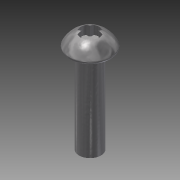
# Autodesk Inventor part: Screw
Saved by Autodesk Inventor 2015 (Build 190159000, 159)
## iProperties
Created: 2016-01-20
Part Number: Screw
Material: Generic
Document SubType Name: Modeling
Designer: Kyle
Density: 1 g/cm^3
Appearance: Galvanized
Author: Kyle
Autodesk Inventor part; units mm, degrees
ref_plane "YZ Plane" through (0, 0, 0) normal (1, 0, 0) x (0, 1, 0)
ref_plane "XZ Plane" through (0, 0, 0) normal (0, 1, 0) x (-1, 0, 0)
ref_plane "XY Plane" through (0, 0, 0) normal (0, 0, 1) x (1, 0, 0)
sketch "Sketch1" plane through (0, 0, 0) normal (0, 0, 1) x (1, 0, 0)
  line L0 (2.1581, 5.715) -> (1.27, 5.715)
  line L1 (1.27, 5.715) -> (1.27, 0)
  line L2 (1.27, 0) -> (0, 0)
  line L3 (0, 0) -> (0, 7.62)
  arc A0 (2.3846, 6.084) -> (0, 7.62) centre (-0.1226, 4.8107) ccw
  arc A1 (2.1581, 5.715) -> (2.3846, 6.084) centre (2.1581, 5.969) ccw
  point P0 (2.54, 5.715)
  dimension "d0" = 7.62
  dimension "d1" = 2.54
  dimension "d2" = 1.905
  dimension "d3" = 1.27
  dimension "d4" = 0.254
  constraints: 8 end point, 5 point on circle, 3 perpendicular, 2 centre point, 2 tangent, 1 horizontal, 1 point on line
  measures "d0" distance of L3.end L2.end
  measures "d1" horizontal distance of point (2.54, 5.715) L3.end
  measures "d2" vertical distance of L3.end point (2.54, 5.715)
  measures "d3" distance of L2.end L1.end
  measures "d4" radius of A1
revolve "Revolution1" add sketch "Sketch1" angle 360 about axis through (0, 0, 0) along (0, 1, 0)
sketch "Sketch2" plane through (0, 0, 0) normal (0, -1, 0) x (1, 0, 0)
  circle A0 centre (0, 0) radius 1.27 projected
  line L0 (0.9525, 0.508) -> (0.508, 0.508)
  line L1 (0.508, 0.508) -> (0.508, 0.9525)
  line L2 (-0.508, 0.9525) -> (-0.508, 0.508)
  line L3 (-0.508, 0.508) -> (-0.9525, 0.508)
  line L4 (-0.9525, -0.508) -> (-0.508, -0.508)
  line L5 (-0.508, -0.508) -> (-0.508, -0.9525)
  line L6 (0.508, -0.9525) -> (0.508, -0.508)
  line L7 (0.9525, -0.508) -> (0.508, -0.508)
  arc A1 (0.9525, -0.508) -> (0.9525, 0.508) centre (0, 0) ccw
  arc A2 (-0.508, -0.9525) -> (0.508, -0.9525) centre (0, 0) ccw
  arc A3 (0.508, 0.9525) -> (-0.508, 0.9525) centre (0, 0) ccw
  arc A4 (-0.9525, 0.508) -> (-0.9525, -0.508) centre (0, 0) ccw
  point P0 (1.164, -0.508)
  point P1 (1.164, 0.508)
  point P2 (-1.164, -0.508)
  point P3 (-1.164, 0.508)
  point P4 (0.508, -1.164)
  point P5 (-0.508, -1.164)
  point P6 (-0.508, 1.164)
  point P7 (0.508, 1.164)
  dimension "d6" = 0.508
  dimension "d7" = 0.508
  constraints: 16 end point, 8 point on circle, 4 centre point, 4 perpendicular, 4 point on line, 2 parallel, 1 coincident, 1 horizontal, 9 other
  measures "d6" vertical distance of point (0, 0) point (1.164, -0.508)
  measures "d7" horizontal distance of point (0, 0) point (0.508, -1.164)
extrude "Extrusion1" cut sketch "Sketch2" against normal blind 25.4 contours A1 L7 L6 A2 L5 L4 A4 L3 L2 A3 L1 L0
sketch "Sketch3" plane through (0, 0, 0) normal (0, -1, 0) x (1, 0, 0)
  circle A0 centre (0, 0) radius 1.27
  constraints: 1 centre point, 1 coincident
extrude "Extrusion2" add sketch "Sketch3" against normal blind 6.35
sketch "Sketch4" plane through (0, 0, 0) normal (0, -1, 0) x (1, 0, 0)
  circle A0 centre (0, 0) radius 1.27
  constraints: 1 centre point, 1 coincident
extrude "Extrusion3" add sketch "Sketch4" along normal blind 4.445
body "Solid1"
